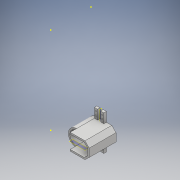
# Autodesk Inventor part: actionneur linéaire
Saved by Autodesk Inventor 2018 (Build 220112000, 112)
## iProperties
Created: 2018-04-06
Part Number: actionneur linéaire
Material: Générique
Document SubType Name: Tôle
Designer: Dimitri
Density: 1 g/cm^3
Appearance: Par défaut
Sheet Metal Rule: Par défaut
Author: Dimitri
Autodesk Inventor part; units mm, degrees
ref_plane "YZ Plane" through (0, 0, 0) normal (1, 0, 0) x (0, 1, 0)
ref_plane "XZ Plane" through (0, 0, 0) normal (0, 1, 0) x (-1, 0, 0)
ref_plane "XY Plane" through (0, 0, 0) normal (0, 0, 1) x (1, 0, 0)
sketch "Esquisse1" plane through (0, 0, 0) normal (0, 1, 0) x (-1, 0, 0)
  line L0 (-61.8861, -256.597) -> (-116.8861, -256.597)
  line L1 (-116.8861, -256.597) -> (-116.8861, -296.597)
  line L2 (-116.8861, -296.597) -> (-61.8861, -296.597)
  arc A0 (-61.8861, -296.597) -> (-61.8861, -256.597) centre (-61.8861, -276.597) ccw
  dimension "d1" = 40
  dimension "d2" = 55
  dimension "d3" = 55
  constraints: 6 end point, 2 perpendicular, 2 point on circle, 1 centre point, 1 horizontal
  measures "d1" distance of L0.end L1.end
  measures "d2" distance of L0.start L0.end
  measures "d3" distance of L1.end L2.end
extrude "Extrusion1" add sketch "Esquisse1" along normal blind 10
sketch "Esquisse3" plane through (0, 0, 0) normal (0, -1, 0) x (1, 0, 0)
  line L0 (89.3861, -269.097) -> (104.3861, -269.097)
  line L1 (104.3861, -269.097) -> (104.3861, -284.097)
  line L2 (104.3861, -284.097) -> (89.3861, -284.097)
  line L3 (89.3861, -284.097) -> (89.3861, -269.097)
  line L4 (116.8861, -296.597) -> (61.8861, -296.597) projected
  line L5 (116.8861, -256.597) -> (116.8861, -296.597) projected
  point P0 (0, 0)
  dimension "d19" = 15
  dimension "d20" = 15
  dimension "d21" = 12.5
  dimension "d22" = 12.5
  constraints: 8 end point, 2 parallel, 1 horizontal, 1 perpendicular
  measures "d19" distance of L0.start L0.end
  measures "d20" distance of L0.end L1.end
  measures "d21" distance between parallel lines of L4 L2
  measures "d22" distance between parallel lines of L5 L1
extrude "Extrusion3" add sketch "Esquisse3" along normal blind 15
chamfer "Chanfrein2" distance 4 angle 45 4 edges at (89.3861, -7.5, -284.097) (104.3861, -7.5, -284.097) (89.3861, -7.5, -269.097) (104.3861, -7.5, -269.097)
sketch "Esquisse4" plane through (0, 10, 0) normal (0, 1, 0) x (1, 0, 0)
  line L0 (116.8861, 296.597) -> (61.8861, 296.597) projected
  arc A0 (61.8861, 296.597) -> (61.8861, 256.597) centre (61.8861, 276.597) ccw projected
  circle A1 centre (61.8861, 276.597) radius 19
  point P0 (0, 0)
  dimension "d28" = 1
  constraints: 1 centre point, 1 coincident, 1 point on circle
  measures "d28" radial gap between concentric circles of A0 A1
extrude "Extrusion4" add sketch "Esquisse4" along normal blind 73
chamfer "Chanfrein3" distance 10 angle 45 2 edges at (116.8861, 5, -256.597) (116.8861, 5, -296.597)
sketch "Esquisse5" plane through (0, 10, 0) normal (0, 1, 0) x (1, 0, 0)
  line L0 (61.8861, 256.597) -> (106.8861, 256.597) projected
  line L1 (106.8861, 296.597) -> (61.8861, 296.597) projected
  arc A0 (97.6044, 288.5312) -> (97.6044, 264.6628) centre (93.8861, 276.597) ccw
  circle A1 centre (61.8861, 276.597) radius 19 projected
  line L2 (116.8861, 266.597) -> (116.8861, 286.597) projected
  line L3 (116.8861, 267.597) -> (116.8861, 285.597)
  line L4 (116.8861, 267.597) -> (93.8861, 264.097)
  line L5 (116.8861, 285.597) -> (93.8861, 289.097)
  point P0 (0, 0)
  dimension "d34" = 25
  dimension "d35" = 32
  dimension "d36" = 1
  dimension "d37" = 1
  constraints: 6 end point, 4 point on circle, 4 point on line, 1 centre point
  measures "d34" diameter of A0
  measures "d35" distance of A1.centre A0.centre
  measures "d36" distance of L2.start L3.start
  measures "d37" distance of L2.end L3.end
extrude "Extrusion5" add sketch "Esquisse5" along normal blind 110 contours L5 L2 L4 A0
sketch "Esquisse6" plane through (0, 120, 0) normal (0, 1, 0) x (1, 0, 0)
  line L0 (116.8861, 267.597) -> (93.8861, 264.097) projected
  arc A0 (93.8861, 289.097) -> (93.8861, 264.097) centre (93.8861, 276.597) ccw projected
  line L1 (93.8861, 264.097) -> (93.8861, 264.097)
  circle A1 centre (93.8861, 276.597) radius 10
  point P0 (0, 0)
  dimension "d40" = 20
  constraints: 2 end point, 1 centre point, 1 coincident, 1 vertical
  measures "d40" diameter of A1
extrude "Extrusion6" add sketch "Esquisse6" along normal blind 22
ref_plane "Plan de construction1" through (61.8861, 0, -276.597) normal (0, 0, -1) x (-1, 0, 0)
sketch "Esquisse7" plane through (61.8861, 0, -276.597) normal (0, 0, -1) x (-1, 0, 0)
  point P0 (61.8861, 0)
sketch "Esquisse8" plane through (0, 0, 0) normal (0, -1, 0) x (1, 0, 0)
  point P0 (0, 0)
sketch "Esquisse9" plane through (0, 0, 0) normal (0, -1, 0) x (1, 0, 0)
  arc A0 (61.8861, -256.597) -> (61.8861, -296.597) centre (61.8861, -276.597) ccw projected
  line L0 (61.8861, -256.597) -> (106.8861, -256.597) projected
  line L1 (106.8861, -256.597) -> (116.8861, -266.597) projected
  line L2 (116.8861, -266.597) -> (116.8861, -286.597) projected
  line L3 (116.8861, -286.597) -> (106.8861, -296.597) projected
  line L4 (106.8861, -296.597) -> (61.8861, -296.597) projected
  line L5 (61.8861, -256.597) -> (106.8861, -256.597) projected
  line L6 (61.8861, -255.597) -> (106.8861, -255.597)
  line L7 (106.8861, -255.597) -> (117.5932, -265.8899)
  line L8 (117.5932, -265.8899) -> (117.5932, -287.3041)
  line L9 (117.5932, -287.3041) -> (106.8861, -297.597)
  line L10 (106.8861, -297.597) -> (61.8861, -297.597)
  arc A1 (61.8861, -255.597) -> (61.8861, -297.597) centre (61.8861, -276.597) ccw
  line L11 (108.8997, -250.597) -> (61.8861, -250.597)
  arc A2 (61.8861, -250.597) -> (61.8861, -302.597) centre (61.8861, -276.597) ccw
  line L12 (61.8861, -302.597) -> (108.8997, -302.597)
  line L13 (108.8997, -302.597) -> (122.5932, -289.4332)
  line L14 (122.5932, -289.4332) -> (122.5932, -263.7609)
  line L15 (122.5932, -263.7609) -> (108.8997, -250.597)
  point P0 (0, 0)
  dimension "d51" = 1
  dimension "d52" = 1
  dimension "d53" = 1
  dimension "d54" = 5
  constraints: 20 end point, 4 point on circle, 2 centre point, 2 perpendicular, 1 coincident, 1 tangent, 1 vertical, 5 other
  measures "d51" distance of L3.end L9.end
  measures "d52" distance of L0.end L6.end
  measures "d53" distance of L1.end L7.end
  measures "d54" distance between parallel lines of L6 L11
extrude "Extrusion7" add sketch "Esquisse9" against normal blind 85 contours L15 L14 L13 L12 A2 L11
sketch "Esquisse10" plane through (0, 0, 0) normal (0, -1, 0) x (1, 0, 0)
  line L0 (89.3861, -273.097) -> (89.3861, -280.097) projected
  line L1 (104.3861, -280.097) -> (104.3861, -273.097) projected
  line L2 (61.8861, -302.597) -> (108.8997, -302.597) projected
  line L3 (89.3861, -250.597) -> (89.3861, -263.7609)
  line L4 (89.3861, -302.597) -> (79.3861, -302.597)
  line L5 (79.3861, -302.597) -> (79.3861, -250.597)
  line L6 (122.5932, -263.7609) -> (89.3861, -263.7609)
  line L7 (89.3861, -268.7609) -> (122.5932, -268.7609)
  line L8 (122.5932, -289.4332) -> (89.3861, -289.4332)
  line L9 (89.3861, -284.4332) -> (122.5932, -284.4332)
  line L10 (89.3861, -289.4332) -> (89.3861, -302.597)
  line L11 (89.3861, -268.7609) -> (89.3861, -284.4332)
  line L12 (79.3861, -250.597) -> (89.3861, -250.597)
  line L13 (108.8997, -250.597) -> (61.8861, -250.597) projected
  line L14 (122.5932, -263.7609) -> (122.5932, -268.7609)
  line L15 (122.5932, -284.4332) -> (122.5932, -289.4332)
  point P0 (0, 0)
  dimension "d57" = 10
  dimension "d58" = 5
  dimension "d59" = 5
  constraints: 24 end point, 9 perpendicular, 3 point on line, 1 collinear, 1 vertical
  measures "d57" distance of L4.start L4.end
  measures "d58" distance of L3.end L7.start
  measures "d59" distance of L8.end L9.start
extrude "Extrusion8" add sketch "Esquisse10" along normal blind 15
sketch "Esquisse11" plane through (0, 85, 0) normal (0, 1, 0) x (1, 0, 0)
  line L0 (116.8861, 286.597) -> (114.0499, 289.4332) projected
  line L1 (116.8861, 286.597) -> (116.8861, 266.597)
  line L2 (61.8861, 256.597) -> (106.8861, 256.597) projected
  line L3 (106.8861, 256.597) -> (61.8861, 256.597)
  line L4 (114.0499, 289.4332) -> (106.8861, 296.597) projected
  line L5 (106.8861, 296.597) -> (61.8861, 296.597)
  line L6 (106.8861, 296.597) -> (61.8861, 296.597) projected
  line L7 (61.8861, 296.597) -> (106.8861, 296.597)
  line L8 (106.8861, 296.597) -> (116.8861, 286.597)
  arc A0 (61.8861, 296.597) -> (61.8861, 256.597) centre (61.8861, 276.597) ccw
  line L9 (114.0499, 263.7609) -> (116.8861, 266.597) projected
  line L10 (116.8861, 266.597) -> (106.8861, 256.597)
  point P0 (0, 0)
  constraints: 12 end point, 3 collinear, 2 point on circle, 1 centre point, 1 horizontal, 1 vertical
extrude "Extrusion9" cut sketch "Esquisse11" against normal blind 85 and the other way blind 42.5
sketch "Esquisse12" plane through (93.8861, 127.5, -276.597) normal (0, -1, 0) x (1, 0, 0)
  point P0 (-93.8861, 276.597)
sketch "Esquisse13" plane through (93.8861, 142, -276.597) normal (0, 1, 0) x (1, 0, 0)
  circle A0 centre (0, 0) radius 10.5
  point P0 (-93.8861, -276.597)
  dimension "d66" = 21
  constraints: 1 centre point
  measures "d66" diameter of A0
extrude "Extrusion10" cut sketch "Esquisse13" against normal blind 85
sketch "Esquisse14" plane through (0, -15, 0) normal (0, -1, 0) x (1, 0, 0)
  line L0 (89.3861, -284.4332) -> (89.3861, -280.097) projected
  line L1 (89.3861, -268.7609) -> (122.5932, -268.7609) projected
  line L2 (89.3861, -284.4332) -> (113.204, -284.4332)
  line L3 (113.204, -284.4332) -> (113.204, -268.7609)
  line L4 (113.204, -268.7609) -> (89.3861, -268.7609)
  line L5 (89.3861, -268.7609) -> (89.3861, -284.4332)
  point P0 (0, 0)
  constraints: 8 end point, 2 parallel, 1 horizontal, 1 perpendicular, 1 point on line
extrude "Extrusion11" cut sketch "Esquisse14" against normal blind 85
sketch "Esquisse17" plane through (61.8861, 85, -250.597) normal (0, 0, 1) x (1, 0, 0)
  line L0 (0, 0) -> (10, 0)
  line L1 (10, 0) -> (10, -8)
  line L2 (10, -8) -> (0, -8)
  line L3 (0, -8) -> (0, 0)
  line L4 (10, 0) -> (20, 0)
  line L5 (0, 0) -> (47.0135, 0) projected
  line L6 (20, 0) -> (30, 0)
  line L7 (30, 0) -> (30, -8)
  line L8 (30, -8) -> (20, -8)
  line L9 (20, -8) -> (20, 0)
  point P0 (-61.8861, -85)
  dimension "d79" = 10
  dimension "d80" = 8
  dimension "d81" = 10
  dimension "d82" = 10
  constraints: 18 end point, 4 parallel, 2 horizontal, 2 perpendicular, 1 point on line
  measures "d79" distance of L1.end L2.end
  measures "d80" distance of L0.end L1.end
  measures "d81" distance of L0.end L4.end
  measures "d82" distance of L7.end L8.end
extrude "Extrusion13" add sketch "Esquisse17" along normal blind 30
sketch "Esquisse18" plane through (81.8861, 77, -250.597) normal (0, -1, 0) x (1, 0, 0)
  line L0 (10, 30) -> (0, 30) projected
  point P0 (-81.8861, 250.597)
  point P1 (5, 22)
  point P2 (5, 10)
ref_plane "Plan de construction2" through (76.8861, 77, -250.597) normal (-1, 0, 0) x (0, 0, 1)
hole "Perçage1" at (86.8861, 77, -240.597) at (86.8861, 77, -228.597) direction (0, 1, 0) diameter 4 end through all
mirror "Symétrie1" about plane through (76.8861, 77, -250.597) normal (-1, 0, 0) of "Perçage1"
mirror "Symétrie2" about plane through (61.8861, 0, -276.597) normal (0, 0, -1) of "Extrusion13", "Perçage1", "Symétrie1"
sketch "Esquisse19" plane through (0, 0, 0) normal (0, -1, 0) x (1, 0, 0)
  line L0 (61.8861, -302.597) -> (79.3861, -302.597) projected
  line L1 (61.8861, -302.597) -> (131.8861, -302.597)
  line L2 (131.8861, -302.597) -> (131.8861, -247.7831)
  line L3 (131.8861, -247.7831) -> (61.8861, -247.7831)
  line L4 (61.8861, -247.7831) -> (61.8861, -302.597)
  point P0 (0, 0)
  point P1 (61.8861, -250.597)
  dimension "d95" = 70
  constraints: 8 end point, 2 parallel, 1 horizontal, 1 perpendicular
  measures "d95" distance of L2.end L3.end
extrude "Extrusion14" cut sketch "Esquisse19" along normal blind 15
sketch "Esquisse20" plane through (0, 0, 0) normal (0, -1, 0) x (1, 0, 0)
  line L0 (61.8861, -250.597) -> (61.8861, -220.597) projected
  arc A0 (61.8861, -255.597) -> (61.8861, -297.597) centre (61.8861, -276.597) ccw projected
  line L1 (61.8861, -250.597) -> (61.8861, -255.597)
  line L2 (61.8861, -297.597) -> (61.8861, -303.2676)
  line L3 (61.8861, -302.597) -> (71.8861, -302.597) projected
  arc A1 (61.8861, -250.597) -> (61.8861, -302.597) centre (61.8861, -276.597) ccw
  arc A2 (61.8861, -255.597) -> (61.8861, -297.597) centre (61.8861, -276.597) ccw
  point P0 (0, 0)
  constraints: 4 end point, 4 point on circle, 2 centre point, 2 coincident, 2 vertical
extrude "Extrusion15" cut sketch "Esquisse20" against normal blind 20
equation "\"d93\" = Epaisseur"
equation "\"RayonPli\" = Epaisseur"
equation "\"LargeurGrugeage\" = Epaisseur"
equation "\"ProfondeurGrugeage\" = 0.5 * Epaisseur"
equation "\"TailleGrugeage\" = 4 * Epaisseur"
equation "\"RestesMinimum\" = 2 * Epaisseur"
equation "\"Rayondetransition\" = RayonPli"
equation "\"TailleRayonJacobi\" = Epaisseur"
equation "\"TailleJeu\" = Epaisseur"
equation "\"Epaisseur\" = 0.5"
